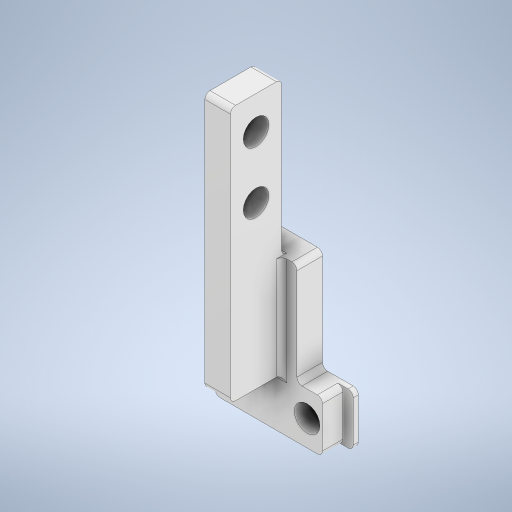
# Autodesk Inventor part: BP_BOX-Support-Bar-Connect1-Right
Saved by Autodesk Inventor 2024.3 (Build 283343000, 343)
## iProperties
Created: 2025-11-18
Part Number: BP_BOX-Support-Bar-Connect1-Right
Material: ABS プラスチック
Document SubType Name: Modeling
Designer: 佐藤智貴
Density: 1.06 g/cm^3
Appearance: 滑らか - 白
Author: 佐藤智貴
Autodesk Inventor part; units mm, degrees
ref_plane "YZ Plane" through (0, 0, 0) normal (1, 0, 0) x (0, 1, 0)
ref_plane "XZ Plane" through (0, 0, 0) normal (0, 1, 0) x (-1, 0, 0)
ref_plane "XY Plane" through (0, 0, 0) normal (0, 0, 1) x (1, 0, 0)
sketch "スケッチ6" plane through (0, 0, 0) normal (0, 0, 1) x (1, 0, 0)
  line L0 (0, 0) -> (25, 0)
  line L1 (25, 0) -> (25, 30)
  line L2 (25, 30) -> (0, 30)
  line L3 (0, 30) -> (0, 0)
  circle A0 centre (5, 5) radius 2.5
  circle A1 centre (20, 5) radius 2.5
  dimension "d39" = 5
  dimension "d40" = 5
  dimension "d41" = 5
  dimension "d42" = 5
  dimension "d43" = 15
  dimension "d44" = 5
  dimension "d45" = 5
  dimension "d46" = 30
  constraints: 8 end point, 2 centre point, 2 parallel, 1 horizontal, 1 perpendicular
  measures "d39" diameter of A0
  measures "d40" diameter of A1
  measures "d41" distance from line of L0 A0.centre
  measures "d42" distance from line of L0 A1.centre
  measures "d43" distance of A1.centre A0.centre
  measures "d44" distance from line of L3 A0.centre
  measures "d45" distance from line of L1 A1.centre
  measures "d46" distance of L0.end L1.end
extrude "押し出し4" add sketch "スケッチ6" along normal blind 5
sketch "スケッチ7" plane through (0, 0, 5) normal (0, 0, 1) x (1, 0, 0)
  line L0 (25, 30) -> (0, 30) projected
  line L1 (10, 30) -> (15, 30)
  line L2 (15, 30) -> (15, 10)
  line L3 (15, 10) -> (10, 10)
  line L4 (10, 10) -> (10, 30)
  line L5 (25, 0) -> (25, 30) projected
  line L6 (0, 30) -> (0, 0) projected
  line L7 (0, 0) -> (25, 0) projected
  line L8 (10, 30) -> (15, 30)
  line L9 (15, 30) -> (15, 60)
  line L10 (15, 60) -> (10, 60)
  line L11 (10, 60) -> (10, 30)
  dimension "d49" = 5
  dimension "d50" = 10
  dimension "d51" = 10
  dimension "d52" = 10
  dimension "d55" = 30
  dimension "d56" = 5
  constraints: 16 end point, 4 parallel, 2 horizontal, 2 perpendicular, 1 point on line
  measures "d49" distance between parallel lines of L4 L2
  measures "d50" distance between parallel lines of L5 L2
  measures "d51" distance between parallel lines of L6 L4
  measures "d52" distance between parallel lines of L7 L3
  measures "d55" distance between parallel lines of L0 L10
  measures "d56" distance of L9.end L10.end
extrude "押し出し5" add sketch "スケッチ7" along normal blind 10 contours L2 L3 L4 L0 | L0 L11 L10 L9
sketch "スケッチ8" plane through (10, 30, 5) normal (-1, 0, 0) x (0, 0, 1)
  line L0 (10, 30) -> (10, -20) projected
  line L1 (0, 30) -> (10, 30) projected
  line L2 (0, -20) -> (10, -20) projected
  point P0 (-5, -30)
  point P1 (5, 11.5)
  point P2 (5, 23.5)
  dimension "d57" = 5
  dimension "d58" = 5
  dimension "d59" = 12
  dimension "d60" = 6.5
  dimension "d61" = 31.5
  measures "d57" distance from line of L0 point (5, 11.5)
  measures "d58" distance from line of L0 point (5, 23.5)
  measures "d59" distance of point (5, 11.5) point (5, 23.5)
  measures "d60" distance from line of L1 point (5, 23.5)
  measures "d61" distance from line of L2 point (5, 11.5)
hole "穴3" at (10, 41.5, 10) at (10, 53.5, 10) direction (1, 0, 0) diameter 5 depth 8
sketch "スケッチ9" plane through (0, 0, 5) normal (0, 0, 1) x (1, 0, 0)
  line L0 (10, 30) -> (0, 30) projected
  line L1 (0, 30) -> (7, 30)
  line L2 (7, 30) -> (7, 10)
  line L3 (7, 10) -> (0, 10)
  line L4 (0, 10) -> (0, 30)
  line L5 (25, 0) -> (25, 30) projected
  line L6 (25, 30) -> (18, 30)
  line L7 (18, 30) -> (18, 10)
  line L8 (18, 10) -> (25, 10)
  line L9 (25, 10) -> (25, 30)
  point P0 (0, 0)
  point P1 (5, 30)
  point P2 (18, 20)
  point P3 (7, 20)
  dimension "d70" = 20
  dimension "d72" = 7
  dimension "d73" = 7
  constraints: 16 end point, 4 parallel, 3 midpoint, 2 horizontal, 2 perpendicular, 1 point on line
  measures "d70" distance from line of point (5, 30) L3
  measures "d72" distance between parallel lines of L4 L2
  measures "d73" distance between parallel lines of L5 L7
extrude "押し出し6" cut sketch "スケッチ9" against normal blind 10
fillet "フィレット4" radius 1 15 edges at (7, 30, 2.5) (12.5, 60, 5) (12.5, 60, 15) (12.5, 10, 15) (7, 10, 2.5) (0, 10, 2.5) (0, 0, 2.5) (18, 30, 2.5) (18, 10, 2.5) (25, 10, 2.5) (25, 0, 2.5) (10, 20, 5) (12.5, 30, 5) (15, 20, 5) (12.5, 10, 5)
sketch "スケッチ10" plane through (0, 0, 5) normal (0, 0, 1) x (1, 0, 0)
  line L0 (9, 30) -> (9, 9) projected
  line L1 (9, 30) -> (8, 30) projected
  arc A0 (8, 30) -> (7, 29) centre (8, 29) ccw projected
  line L2 (7, 29) -> (7, 11) projected
  arc A1 (6, 10) -> (7, 11) centre (6, 11) ccw projected
  line L3 (6, 10) -> (1, 10) projected
  arc A2 (1, 10) -> (0, 9) centre (1, 9) ccw projected
  line L4 (0, 9) -> (0, 1) projected
  arc A3 (0, 1) -> (1, 0) centre (1, 1) ccw projected
  line L5 (1, 0) -> (24, 0) projected
  arc A4 (24, 0) -> (25, 1) centre (24, 1) ccw projected
  line L6 (25, 1) -> (25, 9) projected
  arc A5 (25, 9) -> (24, 10) centre (24, 9) ccw projected
  line L7 (24, 10) -> (19, 10) projected
  arc A6 (18, 11) -> (19, 10) centre (19, 11) ccw projected
  line L8 (18, 11) -> (18, 29) projected
  arc A7 (18, 29) -> (17, 30) centre (17, 29) ccw projected
  line L9 (17, 30) -> (16, 30) projected
  line L10 (16, 9) -> (16, 30) projected
  line L11 (9, 9) -> (16, 9) projected
  circle A8 centre (5, 5) radius 2.5 projected
  circle A9 centre (20, 5) radius 2.5 projected
  line L12 (2, 8) -> (23, 8)
  line L13 (23, 8) -> (23, 2)
  line L14 (23, 2) -> (2, 2)
  line L15 (2, 2) -> (2, 8)
  line L16 (2, 10) -> (2, 0)
  line L17 (24, 10) -> (19, 10) projected
  line L18 (23, 10) -> (23, 0)
  point P0 (0, 0)
  point P1 (2, 2)
  point P2 (23, 2)
  dimension "d77" = 2
  dimension "d78" = 2
  dimension "d79" = 2
  dimension "d80" = 2
  constraints: 12 end point, 4 point on line, 2 parallel, 2 perpendicular, 1 horizontal, 1 vertical
  measures "d77" distance between parallel lines of L5 L14
  measures "d78" distance between parallel lines of L3 L12
  measures "d79" distance between parallel lines of L4 L15
  measures "d80" distance between parallel lines of L6 L13
extrude "押し出し7" cut sketch "スケッチ10" against normal blind 4 contours L16 L15 L5 A3 L4 A2 L3 | L18 L7 A5 L6 A4 L5 L13
fillet "フィレット5" radius 1 4 edges at (23, 10, 3) (23, 0, 3) (2, 10, 3) (2, 0, 3)
equation "\"d42\" = d41"
equation "\"d45\" = d44"
equation "\"d58\" = d57"
equation "\"d73\" = d72"
